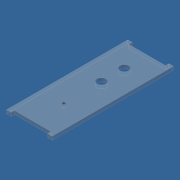
# Autodesk Inventor part: S1702_paroiinterne
Saved by Autodesk Inventor 2015 SP2 (Build 190223200, 223)
## iProperties
Created: 2017-10-31
Part Number: S1702_paroiinterne
Project: S1702_Circuit_Course
Material: Plastique PMMA
Description: Paroi Interne Replat
Document SubType Name: Modeling
Designer: Benoit.CURCHOD2
Authority: 106x40x3
Density: 1.188 g/cm^3
Appearance: Transparent - Clair
Mass: 14.0695 g
Surface Area: 89.7757 cm^2
Volume: 11.8431 cm^3
Material number: ---
Author: Benoit.CURCHOD2
Autodesk Inventor part; units mm, degrees
ref_plane "Plan YZ" through (0, 0, 0) normal (1, 0, 0) x (0, 1, 0)
ref_plane "Plan XZ" through (0, 0, 0) normal (0, 1, 0) x (-1, 0, 0)
ref_plane "Plan XY" through (0, 0, 0) normal (0, 0, 1) x (1, 0, 0)
sketch "Esquisse1" plane through (0, 0, 0) normal (0, 0, 1) x (1, 0, 0)
  line L0 (4, 3) -> (36, 3)
  line L1 (36, 103) -> (4, 103)
  line L2 (0, 106) -> (4, 106)
  line L3 (4, 106) -> (4, 103)
  line L4 (40, 106) -> (36, 106)
  line L5 (36, 106) -> (36, 103)
  line L6 (0, 0) -> (4, 0)
  line L7 (4, 0) -> (4, 3)
  line L8 (36, 3) -> (36, 0)
  line L9 (36, 0) -> (40, 0)
  line L10 (40, 0) -> (40, 106)
  line L11 (0, 0) -> (0, 106)
  dimension "d6" = 100
  dimension "d8" = 3
  dimension "d9" = 3
  dimension "d13" = 40
  dimension "d14" = 4
  dimension "d15" = 4
  constraints: 24 end point, 3 collinear, 3 parallel, 2 horizontal, 2 perpendicular, 2 point on line, 2 vertical, 1 coincident
  measures "d6" distance between parallel lines of L0 L1
  measures "d8" distance between parallel lines of L0 L9
  measures "d9" distance between parallel lines of L4 L1
  measures "d13" distance between parallel lines of L10 L11
  measures "d14" distance between parallel lines of L10 L8
  measures "d15" distance between parallel lines of L11 L7
extrude "Extrusion1" add sketch "Esquisse1" along normal blind 3
sketch "Esquisse6" plane through (0, 0, 3) normal (0, 0, 1) x (1, 0, 0)
  line L0 (0, 106) -> (0, 0) projected
  line L1 (40, 0) -> (40, 106) projected
  line L2 (0, -646.5316) -> (20, -646.5316) construction
  line L3 (40, -683.5995) -> (20, -683.5995) construction
  line L4 (20, 88.2545) -> (20, 14.0947) construction
  circle A0 centre (20, 83) radius 3.9
  circle A1 centre (20, 63) radius 3.9
  line L5 (36, 103) -> (4, 103) projected
  line L6 (36, 0) -> (40, 0) projected
  dimension "d18" = 20
  dimension "d19" = 20
  dimension "d20" = 7.8
  dimension "d21" = 7.8
  constraints: 6 end point, 6 point on line, 2 centre point, 2 horizontal, 1 parallel, 1 vertical
  measures "d18" distance of A1.centre A0.centre
  measures "d19" distance from line of L5 A0.centre
  measures "d20" diameter of A0
  measures "d21" diameter of A1
extrude "Extrusion2" cut sketch "Esquisse6" against normal through all
sketch "Esquisse7" plane through (0, 0, 3) normal (0, 0, 1) x (1, 0, 0)
  line L0 (40, 0) -> (40, 106) construction
  line L1 (0, 106) -> (0, 0) construction
  line L2 (20, 50.9423) -> (20, 15.6231) construction
  line L3 (0, 42.5223) -> (20, 42.5223) construction
  line L4 (20, 46.099) -> (40, 46.099) construction
  line L5 (36, 0) -> (40, 0) projected
  point P0 (20, 30)
  dimension "d27" = 30
  constraints: 6 end point, 5 point on line, 2 parallel, 1 perpendicular, 1 vertical
  measures "d27" distance from line of L5 point (20, 30)
hole "Perçage1" at (20, 30, 3) direction (0, 0, -1) diameter 2.459 end through all thread size "M3x0.5" class "6H" standard "ISO M"
